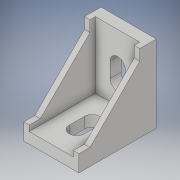
# Autodesk Inventor part: 2020-90
Saved by Autodesk Inventor 2019 (Build 230136000, 136)
## iProperties
Created: 2019-04-21
Part Number: 2020-90
Material: Generic
Document SubType Name: Modeling
Designer: Alex Jones
Density: 1 g/cm^3
Appearance: Default
Author: Alex Jones
Autodesk Inventor part; units mm, degrees
ref_plane "YZ Plane" through (0, 0, 0) normal (1, 0, 0) x (0, 1, 0)
ref_plane "XZ Plane" through (0, 0, 0) normal (0, 1, 0) x (-1, 0, 0)
ref_plane "XY Plane" through (0, 0, 0) normal (0, 0, 1) x (1, 0, 0)
sketch "Sketch1" plane through (0, 0, 0) normal (0, 1, 0) x (-1, 0, 0)
  line L0 (-10, 14) -> (10, 14)
  line L1 (10, 14) -> (10, -14)
  line L2 (10, -14) -> (-10, -14)
  line L3 (-10, -14) -> (-10, 14)
  line L4 (-10, 14) -> (10, -14) construction
  line L5 (10, 14) -> (-10, -14) construction
  point P0 (0, 0)
  dimension "d0" = 28
  dimension "d1" = 20
  constraints: 12 end point, 2 midpoint, 2 parallel, 1 horizontal, 1 perpendicular
  measures "d0" distance of L0.end L1.end
  measures "d1" distance of L0.start L0.end
extrude "Extrusion1" add sketch "Sketch1" along normal blind 4
sketch "Sketch2" plane through (0, 4, 0) normal (0, 1, 0) x (1, 0, 0)
  line L0 (10, 14) -> (-10, 14) projected
  line L1 (-10, 14) -> (10, 14)
  line L2 (10, 14) -> (10, 10)
  line L3 (10, 10) -> (-10, 10)
  line L4 (-10, 10) -> (-10, 14)
  point P0 (0, 0)
  dimension "d4" = 4
  constraints: 8 end point, 2 parallel, 1 horizontal, 1 perpendicular
  measures "d4" distance between parallel lines of L0 L3
extrude "Extrusion2" add sketch "Sketch2" along normal blind 24
sketch "Sketch3" plane through (0, 4, 0) normal (0, 1, 0) x (1, 0, 0)
  line L0 (-10, 10) -> (10, 10) projected
  line L1 (10, -14) -> (8, -14)
  line L2 (8, -14) -> (8, 10)
  line L3 (8, 10) -> (10, 10)
  line L4 (10, 10) -> (10, -14)
  line L5 (-10, -14) -> (-8, -14)
  line L6 (-8, -14) -> (-8, 10)
  line L7 (-8, 10) -> (-10, 10)
  line L8 (-10, 10) -> (-10, -14)
  point P0 (0, 0)
  dimension "d7" = 2
  dimension "d8" = 2
  constraints: 16 end point, 4 parallel, 2 horizontal, 2 perpendicular, 2 point on line
  measures "d7" distance between parallel lines of L4 L2
  measures "d8" distance between parallel lines of L8 L6
extrude "Extrusion3" add sketch "Sketch3" along normal blind 24
sketch "Sketch4" plane through (10, 0, 14) normal (1, 0, 0) x (0, 0, -1)
  line L0 (0, 4) -> (0, 28) projected
  line L1 (24, 28) -> (24, 4) projected
  line L2 (0, 28) -> (24, 28)
  line L3 (24, 28) -> (24, 4)
  line L4 (24, 4) -> (0, 4)
  line L5 (0, 4) -> (0, 28)
  line L6 (0, 28) -> (22, 28)
  line L7 (22, 28) -> (22, 6)
  line L8 (22, 6) -> (0, 6)
  line L9 (0, 6) -> (0, 28)
  line L10 (4, 6) -> (22, 24)
  point P0 (14, 0)
  dimension "d11" = 2
  dimension "d12" = 2
  dimension "d13" = 4
  dimension "d14" = 4
  constraints: 18 end point, 4 parallel, 2 horizontal, 2 perpendicular, 2 point on line
  measures "d11" distance between parallel lines of L4 L8
  measures "d12" distance between parallel lines of L1 L7
  measures "d13" distance from line of L0 L10.start
  measures "d14" distance from line of L2 L10.end
extrude "Extrusion4" cut sketch "Sketch4" against normal blind 24 contours L0 L2 L7 L10 L8
sketch "Sketch5" plane through (0, 4, 0) normal (0, 1, 0) x (1, 0, 0)
  line L0 (-8, -14) -> (8, -14) projected
  line L1 (0, -14) -> (0, 10)
  line L2 (-8, 10) -> (8, 10) projected
  line L3 (2.75, -4.75) -> (-2.75, -4.75)
  line L4 (-2.75, -4.75) -> (-2.75, 0.75)
  line L5 (-2.75, 0.75) -> (2.75, 0.75)
  line L6 (2.75, 0.75) -> (2.75, -4.75)
  line L7 (2.75, -4.75) -> (-2.75, 0.75) construction
  line L8 (-2.75, -4.75) -> (2.75, 0.75) construction
  arc A0 (2.75, 0.75) -> (-2.75, 0.75) centre (0, 0.75) ccw
  arc A1 (-2.75, -4.75) -> (2.75, -4.75) centre (0, -4.75) ccw
  point P0 (0, 0)
  point P1 (0, -2)
  dimension "d17" = 5.5
  dimension "d18" = 5.5
  constraints: 14 end point, 7 midpoint, 4 point on circle, 2 centre point, 2 parallel, 1 horizontal, 1 perpendicular
  measures "d17" distance of L4.end L5.end
  measures "d18" distance between parallel lines of L5 L3
extrude "Extrusion5" cut sketch "Sketch5" against normal blind 24
sketch "Sketch6" plane through (-8, 4, -10) normal (0, 0, 1) x (1, 0, 0)
  line L0 (0, 24) -> (16, 24) projected
  line L1 (8, 24) -> (8, -4)
  line L2 (10.75, 7.25) -> (5.25, 7.25)
  line L3 (5.25, 7.25) -> (5.25, 12.75)
  line L4 (5.25, 12.75) -> (10.75, 12.75)
  line L5 (10.75, 12.75) -> (10.75, 7.25)
  line L6 (10.75, 7.25) -> (5.25, 12.75) construction
  line L7 (5.25, 7.25) -> (10.75, 12.75) construction
  arc A0 (10.75, 12.75) -> (5.25, 12.75) centre (8, 12.75) ccw
  arc A1 (5.25, 7.25) -> (10.75, 7.25) centre (8, 7.25) ccw
  point P0 (8, 10)
  dimension "d21" = 5.5
  dimension "d22" = 5.5
  constraints: 14 end point, 6 midpoint, 4 point on circle, 2 centre point, 2 parallel, 1 horizontal, 1 perpendicular, 1 vertical
  measures "d21" distance of L3.end L4.end
  measures "d22" distance of L4.end L2.start
extrude "Extrusion6" cut sketch "Sketch6" against normal blind 24
body "Solid1"
